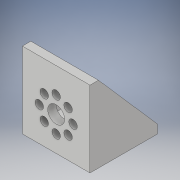
# Autodesk Inventor part: KB33-046-001-002 - Уголок
Saved by Autodesk Inventor 2019 (Build 230136000, 136)
## iProperties
Created: 2021-06-09
Part Number: KB33-046-001-002 - Уголок
Material: Типовые
Document SubType Name: Modeling
Designer: Петров Иван
Density: 1 g/cm^3
Appearance: По умолчанию
Author: Петров Иван
Autodesk Inventor part; units mm, degrees
ref_plane "YZ Plane" through (0, 0, 0) normal (1, 0, 0) x (0, 1, 0)
ref_plane "XZ Plane" through (0, 0, 0) normal (0, 1, 0) x (-1, 0, 0)
ref_plane "XY Plane" through (0, 0, 0) normal (0, 0, 1) x (1, 0, 0)
sketch "Sketch1" plane through (0, 0, 0) normal (0, 1, 0) x (-1, 0, 0)
  line L0 (-16, 16) -> (16, 16)
  line L1 (16, 16) -> (16, -16)
  line L2 (16, -16) -> (-16, -16)
  line L3 (-16, -16) -> (-16, 16)
  line L4 (-16, 16) -> (16, -16) construction
  line L5 (16, 16) -> (-16, -16) construction
  circle A0 centre (0, 0) radius 4
  dimension "d0" = 32
  dimension "d1" = 32
  dimension "d2" = 8
  constraints: 12 end point, 2 midpoint, 2 parallel, 1 centre point, 1 coincident, 1 horizontal, 1 perpendicular
  measures "d0" distance of L1.end L2.end
  measures "d1" distance of L0.end L1.end
  measures "d2" diameter of A0
extrude "Extrusion1" add sketch "Sketch1" along normal blind 4
sketch "Sketch2" plane through (0, 4, 0) normal (0, 1, 0) x (1, 0, 0)
  circle A0 centre (-8, 0) radius 2
  point P0 (0, 0)
  dimension "d5" = 4
  dimension "d6" = 8
  constraints: 1 centre point
  measures "d5" diameter of A0
  measures "d6" distance of point (0, 0) A0.centre
extrude "Extrusion2" cut sketch "Sketch2" against normal blind 4
pattern_circular "Circular Pattern1" count 4 over 360 about axis through (0, 0, 0) along (0, 1, 0) of "Extrusion2"
sketch "Sketch3" plane through (0, 4, 0) normal (0, 1, 0) x (1, 0, 0)
  line L0 (-16, -16) -> (-16, 16) projected
  line L1 (-16, -16) -> (16, -16)
  line L2 (16, -16) -> (16, -12)
  line L3 (16, -12) -> (-16, -12)
  line L4 (-16, -12) -> (-16, -16)
  point P0 (0, 0)
  dimension "d12" = 32
  dimension "d13" = 4
  constraints: 8 end point, 2 parallel, 1 horizontal, 1 perpendicular
  measures "d12" distance of L3.end L2.end
  measures "d13" distance of L2.end L1.end
extrude "Extrusion3" add sketch "Sketch3" along normal blind 32
sketch "Sketch4" plane through (16, 4, 12) normal (0, 0, -1) x (-1, 0, 0)
  line L0 (32, 0) -> (32, 32) construction
  line L1 (0, 0) -> (0, 32) construction
  circle A0 centre (16, 12) radius 4
  point P0 (16, -4)
  dimension "d16" = 8
  dimension "d26" = 32
  dimension "d27" = 12
  constraints: 1 centre point
  measures "d16" diameter of A0
  measures "d26" distance of L0.start L0.end
  measures "d27" vertical distance of L0.start A0.centre
extrude "Extrusion4" cut sketch "Sketch4" against normal blind 28
sketch "Sketch5" plane through (16, 4, 12) normal (0, 0, -1) x (-1, 0, 0)
  circle A0 centre (24, 12) radius 2
  circle A1 centre (16, 12) radius 4 projected
  point P0 (16, -4)
  dimension "d19" = 4
  dimension "d20" = 8
  constraints: 1 centre point, 1 horizontal alignment
  measures "d19" diameter of A0
  measures "d20" distance of A1.centre A0.centre
extrude "Extrusion5" cut sketch "Sketch5" against normal blind 28 contours A0
pattern_circular "Circular Pattern2" count 8 over 360 about axis through (0, 16, 12) along (0, 0, 1) of "Extrusion5"
sketch "Sketch6" plane through (16, 0, 16) normal (1, 0, 0) x (0, 0, -1)
  line L0 (4, 4) -> (4, 36) projected
  line L1 (32, 0) -> (32, 4) projected
  line L2 (4, 36) -> (32, 4)
  line L3 (4, 4) -> (32, 4) projected
  point P0 (16, 0)
  constraints: 2 end point
extrude "Extrusion6" add sketch "Sketch6" against normal blind 3
mirror "Mirror1" about plane through (0, 0, 0) normal (1, 0, 0) of "Extrusion6"
body "Solid1"
